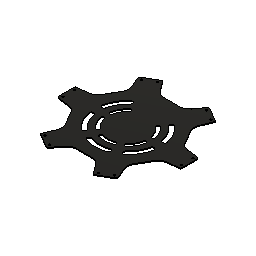
F550 Bottom Plate Type 2 v2 (Autodesk Fusion 360 design; units mm, degrees)
Autodesk Fusion 360 part; units mm, degrees
sketch "Sketch1" plane through (0, 0, 0) normal (0, 0, 1) x (1, 0, 0)
  circle A0 centre (0, 0) radius 275 construction
  line L0 (-110, -15.85) -> (-110, 15.85)
  circle A1 centre (-105, 10.5) radius 1.75
  circle A2 centre (-105, -10.5) radius 1.75
  line L1 (-105, 10.5) -> (-105, -10.5) construction
  line L2 (0, 0) -> (-67.55, 39)
  line L3 (0, 0) -> (-67.55, -39)
  line L4 (0, 0) -> (-105, 0) construction
  line L5 (-110, -15.85) -> (-87.3994, -18.594)
  line L6 (-67.55, -39) -> (-74.3532, -27.2164)
  arc A3 (-74.3532, -27.2164) -> (-87.3994, -18.594) centre (-89.5087, -35.9664) ccw
  line L7 (-110, 15.85) -> (-87.3994, 18.594)
  arc A4 (-87.3994, 18.594) -> (-74.3532, 27.2164) centre (-89.5087, 35.9664) ccw
  line L8 (-67.55, 39) -> (-74.3532, 27.2164)
  point P0 (-110, 0)
  point P1 (-105, 0)
  point P2 (-275, 0)
  point P3 (-107, -10)
  point P4 (-107, 10)
  point P5 (-107, 0)
  dimension "d1" = 550
  dimension "d2" = 21
  dimension "d3" = 5
  dimension "d5" = 170
  dimension "d6" = 3.5
  dimension "d7" = 31.7
  dimension "d8" = 30
  dimension "d9" = 30
  dimension "d10" = 78
  dimension "d13" = 20
  dimension "d30" = 105
  dimension "d56" = 17.5
  constraint coincident A0.centre L2.start
  constraint vertical L0
  constraint midpoint L0 P0
  constraint horizontal A0.centre P0
  constraint vertical A1.centre A2.centre
  constraint coincident A1.centre L1.start
  constraint coincident A2.centre L1.end
  constraint midpoint L1 P1
  constraint coincident A0 P2
  constraint horizontal A0.centre P2
  constraint equal A1 A2
  constraint coincident P1 L4.end
  constraint horizontal A0.centre P1
  constraint equal L2 L3
  constraint perpendicular L3 L6
  constraint tangent L6 A3
  constraint tangent L5 A3
  constraint symmetric L0.start L4 L0.end
  constraint symmetric L3.end L4 L2.end
  constraint symmetric L4 L5.end L7.end
  constraint symmetric L4 L6.end A4.end
  constraint symmetric L4 A3 A4
  constraint coincident L4 P5
  measures "d1" diameter of A0
  measures "d2" distance of A1.centre A2.centre
  measures "d3" distance of L0 L1
  measures "d5" distance of L1 P2
  measures "d6" diameter of A1
  measures "d7" distance of L0.start L0.end
  measures "d8" angle of L3 L4
  measures "d9" angle of L2 L4
  measures "d10" distance of A0.centre L2.end
  measures "d13" distance of P3 P4
  measures "d30" distance of L1 A0.centre
  measures "d56" radius of A4
extrude "Extrude1" add sketch "Sketch1" along normal blind 1.5 makes body 1
fillet "Fillet1" radius 2 2 edges at (-110, 15.85, 0.75) (-110, -15.85, 0.75) on bodies 1
pattern_circular "C-Pattern1" count 6 over 360 about axis through (0, 0, 1.75) along (0, 0, 1) of bodies 1 makes body 2 at (-25.2134, -43.671, 0) makes body 3 at (25.2134, -43.671, 0) makes body 4 at (50.4269, 0, 0) makes body 5 at (25.2134, 43.671, 0) makes body 6 at (-25.2134, 43.671, 0)
combine "Combine1" operation add target body 1 tool bodies 2 3 4 5 6
sketch "Sketch3" plane through (0, 0, 1.5) normal (0, 0, 1) x (-1, 0, 0)
  circle A0 centre (61.5933, -85.6827) radius 1.75
  circle A1 centre (43.4067, -96.1827) radius 1.75
  circle A2 centre (-43.4067, -96.1827) radius 1.75
  circle A3 centre (-61.5933, -85.6827) radius 1.75
  circle A4 centre (-105, -10.5) radius 1.75
  circle A5 centre (-105, 10.5) radius 1.75
  circle A6 centre (-61.5933, 85.6827) radius 1.75
  circle A7 centre (-43.4067, 96.1827) radius 1.75
  circle A8 centre (43.4067, 96.1827) radius 1.75
  circle A9 centre (61.5933, 85.6827) radius 1.75
  arc A10 (110, 14.0781) -> (108.2411, 16.0636) centre (108, 14.0781) ccw
  line L0 (108.2411, 16.0636) -> (87.3994, 18.594)
  arc A11 (74.3532, 27.2164) -> (87.3994, 18.594) centre (89.5087, 35.9664) ccw
  arc A12 (59.8026, 66.3931) -> (60.7467, 50.7836) centre (75.9022, 59.5336) ccw
  line L1 (59.8026, 66.3931) -> (68.032, 85.7077)
  arc A13 (68.032, 85.7077) -> (67.192, 88.2237) centre (66.192, 86.4917) ccw
  line L2 (67.192, 88.2237) -> (42.808, 102.3019)
  arc A14 (42.808, 102.3019) -> (40.2091, 101.7713) centre (41.808, 100.5698) ccw
  line L3 (40.2091, 101.7713) -> (27.5968, 84.9871)
  arc A15 (13.6065, 78) -> (27.5968, 84.9871) centre (13.6065, 95.5) ccw
  line L4 (13.6065, 78) -> (-13.6065, 78)
  arc A16 (-27.5968, 84.9871) -> (-13.6065, 78) centre (-13.6065, 95.5) ccw
  line L5 (-27.5968, 84.9871) -> (-40.2091, 101.7713)
  arc A17 (-40.2091, 101.7713) -> (-42.808, 102.3019) centre (-41.808, 100.5698) ccw
  line L6 (-42.808, 102.3019) -> (-67.192, 88.2237)
  arc A18 (-67.192, 88.2237) -> (-68.032, 85.7077) centre (-66.192, 86.4917) ccw
  line L7 (-68.032, 85.7077) -> (-59.8026, 66.3931)
  arc A19 (-60.7467, 50.7836) -> (-59.8026, 66.3931) centre (-75.9022, 59.5336) ccw
  line L8 (-60.7467, 50.7836) -> (-74.3532, 27.2164)
  arc A20 (-87.3994, 18.594) -> (-74.3532, 27.2164) centre (-89.5087, 35.9664) ccw
  line L9 (-87.3994, 18.594) -> (-108.2411, 16.0636)
  arc A21 (-108.2411, 16.0636) -> (-110, 14.0781) centre (-108, 14.0781) ccw
  line L10 (-110, 14.0781) -> (-110, -14.0781)
  arc A22 (-110, -14.0781) -> (-108.2411, -16.0636) centre (-108, -14.0781) ccw
  line L11 (-108.2411, -16.0636) -> (-87.3994, -18.594)
  arc A23 (-74.3532, -27.2164) -> (-87.3994, -18.594) centre (-89.5087, -35.9664) ccw
  line L12 (-74.3532, -27.2164) -> (-60.7467, -50.7836)
  arc A24 (-59.8026, -66.3931) -> (-60.7467, -50.7836) centre (-75.9022, -59.5336) ccw
  line L13 (-59.8026, -66.3931) -> (-68.032, -85.7077)
  arc A25 (-68.032, -85.7077) -> (-67.192, -88.2237) centre (-66.192, -86.4917) ccw
  line L14 (-67.192, -88.2237) -> (-42.808, -102.3019)
  arc A26 (-42.808, -102.3019) -> (-40.2091, -101.7713) centre (-41.808, -100.5698) ccw
  line L15 (-40.2091, -101.7713) -> (-27.5968, -84.9871)
  arc A27 (-13.6065, -78) -> (-27.5968, -84.9871) centre (-13.6065, -95.5) ccw
  line L16 (-13.6065, -78) -> (13.6065, -78)
  arc A28 (27.5968, -84.9871) -> (13.6065, -78) centre (13.6065, -95.5) ccw
  line L17 (27.5968, -84.9871) -> (40.2091, -101.7713)
  arc A29 (40.2091, -101.7713) -> (42.808, -102.3019) centre (41.808, -100.5698) ccw
  line L18 (42.808, -102.3019) -> (67.192, -88.2237)
  arc A30 (67.192, -88.2237) -> (68.032, -85.7077) centre (66.192, -86.4917) ccw
  line L19 (68.032, -85.7077) -> (59.8026, -66.3931)
  arc A31 (60.7467, -50.7836) -> (59.8026, -66.3931) centre (75.9022, -59.5336) ccw
  arc A32 (87.3994, -18.594) -> (74.3532, -27.2164) centre (89.5087, -35.9664) ccw
  line L20 (87.3994, -18.594) -> (108.2411, -16.0636)
  arc A33 (108.2411, -16.0636) -> (110, -14.0781) centre (108, -14.0781) ccw
  line L21 (110, -14.0781) -> (110, 14.0781)
  circle A34 centre (105, -10.5) radius 1.75
  circle A35 centre (105, 10.5) radius 1.75
  arc A36 (27.2352, -30.5131) -> (40.0428, -8.3298) centre (0, 0) ccw
  arc A37 (23.373, -26.1861) -> (27.2352, -30.5131) centre (25.3041, -28.3496) ccw
  arc A38 (23.373, -26.1861) -> (34.3643, -7.1486) centre (0, 0) ccw
  arc A39 (40.0428, -8.3298) -> (34.3643, -7.1486) centre (37.2036, -7.7392) ccw
  arc A40 (25.3041, -28.3496) -> (37.2036, -7.7392) centre (0, 0) ccw construction
  arc A41 (39.17, -43.8538) -> (57.5635, -11.9953) centre (0, 0) ccw
  arc A42 (34.1072, -38.1856) -> (39.17, -43.8538) centre (36.6386, -41.0197) ccw
  arc A43 (34.1072, -38.1856) -> (50.1233, -10.4449) centre (0, 0) ccw
  arc A44 (57.5635, -11.9953) -> (50.1233, -10.4449) centre (53.8434, -11.2201) ccw
  arc A45 (36.6386, -41.0197) -> (53.8434, -11.2201) centre (0, 0) ccw construction
  line L22 (0, 0) -> (55, -95.2628) construction
  line L23 (0, 0) -> (110, 0) construction
  arc A46 (53.8434, 11.2201) -> (36.6386, 41.0197) centre (0, 0) ccw construction
  arc A47 (37.2036, 7.7392) -> (25.3041, 28.3496) centre (0, 0) ccw construction
  arc A48 (40.0428, 8.3298) -> (27.2352, 30.5131) centre (0, 0) ccw
  arc A49 (57.5635, 11.9953) -> (39.17, 43.8538) centre (0, 0) ccw
  arc A50 (34.3643, 7.1486) -> (23.373, 26.1861) centre (0, 0) ccw
  arc A51 (50.1233, 10.4449) -> (34.1072, 38.1856) centre (0, 0) ccw
  arc A52 (39.17, 43.8538) -> (34.1072, 38.1856) centre (36.6386, 41.0197) ccw
  arc A53 (50.1233, 10.4449) -> (57.5635, 11.9953) centre (53.8434, 11.2201) ccw
  arc A54 (27.2352, 30.5131) -> (23.373, 26.1861) centre (25.3041, 28.3496) ccw
  arc A55 (34.3643, 7.1486) -> (40.0428, 8.3298) centre (37.2036, 7.7392) ccw
  arc A56 (17.2048, 52.2398) -> (-17.2048, 52.2398) centre (0, 0) ccw construction
  arc A57 (11.8994, 36.0888) -> (-11.8994, 36.0888) centre (0, 0) ccw construction
  arc A58 (12.8075, 38.843) -> (-12.8075, 38.843) centre (0, 0) ccw
  arc A59 (18.3935, 55.8491) -> (-18.3935, 55.8491) centre (0, 0) ccw
  arc A60 (10.9913, 33.3347) -> (-10.9913, 33.3347) centre (0, 0) ccw
  arc A61 (16.0161, 48.6305) -> (-16.0161, 48.6305) centre (0, 0) ccw
  arc A62 (-18.3935, 55.8491) -> (-16.0161, 48.6305) centre (-17.2048, 52.2398) ccw
  arc A63 (16.0161, 48.6305) -> (18.3935, 55.8491) centre (17.2048, 52.2398) ccw
  arc A64 (-12.8075, 38.843) -> (-10.9913, 33.3347) centre (-11.8994, 36.0888) ccw
  arc A65 (10.9913, 33.3347) -> (12.8075, 38.843) centre (11.8994, 36.0888) ccw
  arc A66 (-36.6386, 41.0197) -> (-53.8434, 11.2201) centre (0, 0) ccw construction
  arc A67 (-25.3041, 28.3496) -> (-37.2036, 7.7392) centre (0, 0) ccw construction
  arc A68 (-27.2352, 30.5131) -> (-40.0428, 8.3298) centre (0, 0) ccw
  arc A69 (-39.17, 43.8538) -> (-57.5635, 11.9953) centre (0, 0) ccw
  arc A70 (-23.373, 26.1861) -> (-34.3643, 7.1486) centre (0, 0) ccw
  arc A71 (-34.1072, 38.1856) -> (-50.1233, 10.4449) centre (0, 0) ccw
  arc A72 (-57.5635, 11.9953) -> (-50.1233, 10.4449) centre (-53.8434, 11.2201) ccw
  arc A73 (-34.1072, 38.1856) -> (-39.17, 43.8538) centre (-36.6386, 41.0197) ccw
  arc A74 (-40.0428, 8.3298) -> (-34.3643, 7.1486) centre (-37.2036, 7.7392) ccw
  arc A75 (-23.373, 26.1861) -> (-27.2352, 30.5131) centre (-25.3041, 28.3496) ccw
  arc A76 (-53.8434, -11.2201) -> (-36.6386, -41.0197) centre (0, 0) ccw construction
  arc A77 (-37.2036, -7.7392) -> (-25.3041, -28.3496) centre (0, 0) ccw construction
  arc A78 (-40.0428, -8.3298) -> (-27.2352, -30.5131) centre (0, 0) ccw
  arc A79 (-57.5635, -11.9953) -> (-39.17, -43.8538) centre (0, 0) ccw
  arc A80 (-34.3643, -7.1486) -> (-23.373, -26.1861) centre (0, 0) ccw
  arc A81 (-50.1233, -10.4449) -> (-34.1072, -38.1856) centre (0, 0) ccw
  arc A82 (-39.17, -43.8538) -> (-34.1072, -38.1856) centre (-36.6386, -41.0197) ccw
  arc A83 (-50.1233, -10.4449) -> (-57.5635, -11.9953) centre (-53.8434, -11.2201) ccw
  arc A84 (-27.2352, -30.5131) -> (-23.373, -26.1861) centre (-25.3041, -28.3496) ccw
  arc A85 (-34.3643, -7.1486) -> (-40.0428, -8.3298) centre (-37.2036, -7.7392) ccw
  point P0 (33.8045, -43.5511)
  point P1 (54.6186, -7.5)
  point P2 (37.7942, -4.9)
  point P3 (23.1406, -30.2807)
  point P4 (54.6186, 7.5)
  point P5 (37.7942, 4.9)
  point P6 (74.3532, 27.2164)
  point P7 (23.1406, 30.2807)
  point P8 (33.8045, 43.5511)
  point P9 (20.8141, 51.0511)
  point P10 (14.6536, 35.1807)
  point P11 (13.6065, 78)
  point P12 (-14.6536, 35.1807)
  point P13 (-20.8141, 51.0511)
  point P14 (-33.8045, 43.5511)
  point P15 (-23.1406, 30.2807)
  point P16 (-60.7467, 50.7836)
  point P17 (-37.7942, 4.9)
  point P18 (-54.6186, 7.5)
  point P19 (-54.6186, -7.5)
  point P20 (-37.7942, -4.9)
  point P21 (-74.3532, -27.2164)
  point P22 (-23.1406, -30.2807)
  point P23 (-33.8045, -43.5511)
  dimension "d57" = 38
  dimension "d58" = 55
  dimension "d59" = 3.8
  dimension "d60" = 2.9
  dimension "d61" = 4.9
  dimension "d62" = 7.5
  dimension "d64" = 4.9
  dimension "d65" = 7.5
  dimension "d67" = 360
  constraint tangent A36 A37
  constraint tangent A37 A38
  constraint tangent A38 A39
  constraint tangent A36 A39
  constraint coincident A36.centre A38.centre
  constraint tangent A41 A42
  constraint tangent A42 A43
  constraint tangent A43 A44
  constraint tangent A41 A44
  constraint midpoint L18 L22.end
  constraint midpoint L21 L23.end
  constraint midpoint A42 P0
  constraint midpoint A44 P1
  constraint midpoint A39 P2
  constraint midpoint A37 P3
  measures "d58" radius of A45
  measures "d59" radius of A42
  measures "d60" radius of A37
  measures "d61" distance of L22 P3
  measures "d62" distance of L22 P0
  measures "d64" distance of L23 P2
  measures "d65" distance of L23 P1
extrude "Extrude3" cut sketch "Sketch3" against normal through all contours A36 A37 A38 A39 | A41 A42 A43 A44 | A48 A50 A54 A55 | A49 A51 A52 A53 | A58 A60 A64 A65 | A59 A61 A62 A63 | A68 A70 A74 A75 | A69 A71 A72 A73 | A78 A80 A84 A85 | A79 A81 A82 A83 bodies 1
equation "d9 = d8"
equation "d10 = ( 156 / 2 ) * 1 mm"
equation "d57 = ( 76 / 2 ) * 1 mm"
equation "d58 = ( 110 / 2 ) * 1 mm"
equation "d59 = ( 7.6 / 2 ) * 1 mm"
equation "d60 = ( 5.8 / 2 ) * 1 mm"
equation "d61 = ( 9.8 / 2 ) * 1 mm"
equation "d62 = ( 15 / 2 ) * 1 mm"
equation "d64 = d61"
equation "d65 = d62"
